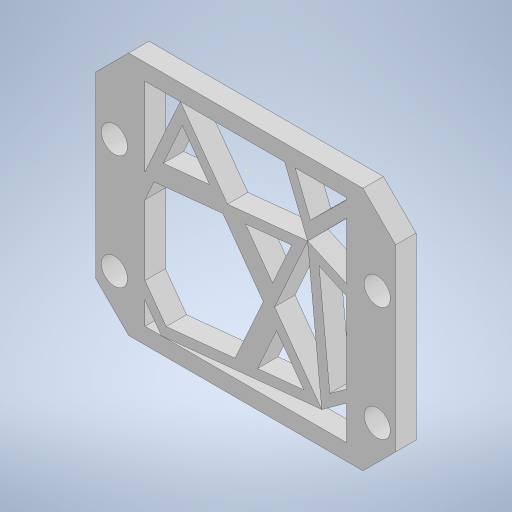
# Autodesk Inventor part: 1министена
Saved by Autodesk Inventor 2023.1 (Build 271208000, 208)
## iProperties
Created: 2025-12-15
Part Number: 1министена
Material: Типовые
Document SubType Name: Modeling
Designer: DELL
Density: 1 g/cm^3
Appearance: По умолчанию
Author: DELL
Autodesk Inventor part; units mm, degrees
ref_plane "YZ Plane" through (0, 0, 0) normal (1, 0, 0) x (0, 1, 0)
ref_plane "XZ Plane" through (0, 0, 0) normal (0, 1, 0) x (-1, 0, 0)
ref_plane "XY Plane" through (0, 0, 0) normal (0, 0, 1) x (1, 0, 0)
sketch "Эскиз1" plane through (0, 0, 0) normal (0, 0, 1) x (1, 0, 0)
  line L0 (18.0359, -24.7333) -> (-18.1641, -24.7333)
  line L1 (-10.3906, -22.7523) -> (-12.4141, -19.9485)
  line L2 (-12.4141, -6.4014) -> (-12.1226, -5.7523)
  line L3 (-12.1226, -5.7523) -> (-2.3077, -4.7523)
  line L4 (-2.3077, -4.7523) -> (3.4658, -12.7523)
  line L5 (3.4658, -12.7523) -> (-0.5756, -21.7523)
  line L6 (-0.5756, -21.7523) -> (-10.3906, -22.7523)
  line L7 (-1.3865, -20.6287) -> (2.0873, -12.8928)
  line L8 (2.0873, -12.8928) -> (-2.8753, -6.0164)
  line L9 (-2.8753, -6.0164) -> (-11.3118, -6.8759)
  line L10 (-11.3118, -6.8759) -> (-12.4141, -9.3307)
  line L11 (-12.4141, -17.8979) -> (-9.823, -21.4883)
  line L12 (-9.823, -21.4883) -> (-1.3865, -20.6287)
  line L13 (-0.5756, -21.7523) -> (9.2393, -20.7523)
  line L14 (9.2393, -20.7523) -> (3.4658, -12.7523)
  line L15 (7.0499, -19.7692) -> (1.3705, -20.3478)
  line L16 (3.7091, -15.14) -> (1.3705, -20.3478)
  line L17 (3.7091, -15.14) -> (7.0499, -19.7692)
  line L18 (-12.1226, -5.7523) -> (-8.0812, 3.2477)
  line L19 (-8.0812, 3.2477) -> (-2.3077, -4.7523)
  line L20 (-2.3077, -4.7523) -> (-12.1226, -5.7523)
  line L21 (-10.1765, -4.3478) -> (-4.4971, -3.7692)
  line L22 (-4.4971, -3.7692) -> (-7.8379, 0.86)
  line L23 (-7.8379, 0.86) -> (-10.1765, -4.3478)
  line L24 (3.4658, -12.7523) -> (-2.3077, -4.7523)
  line L25 (-2.3077, -4.7523) -> (7.5073, -3.7523)
  line L26 (7.5073, -3.7523) -> (3.4658, -12.7523)
  line L27 (-0.1183, -5.7355) -> (5.5611, -5.1568)
  line L28 (5.5611, -5.1568) -> (3.2226, -10.3647)
  line L29 (-0.1183, -5.7355) -> (3.2226, -10.3647)
  line L30 (7.5073, -3.7523) -> (4.6974, 3.2477)
  line L31 (12.2859, 1.0617) -> (7.5073, -3.7523)
  line L32 (12.2859, 3.0053) -> (7.8466, -1.3764)
  line L33 (7.8466, -1.3764) -> (5.9905, 3.2477)
  line L34 (7.5073, -3.7523) -> (9.2393, -20.7523)
  line L35 (9.2393, -20.7523) -> (11.4529, -19.1548)
  line L36 (7.5073, -3.7523) -> (12.2859, -5.8982)
  line L37 (8.9118, -5.6985) -> (12.2859, -7.2136)
  line L38 (10.2225, -18.5629) -> (12.2859, -17.0738)
  line L39 (8.9118, -5.6985) -> (10.2225, -18.5629)
  line L40 (-5.1674, 3.2477) -> (-5.2923, 2.7696)
  line L41 (-5.2923, 2.7696) -> (-7.3317, 2.2091)
  line L42 (-9.7892, 3.2477) -> (-8.6058, 2.0793)
  line L43 (-18.1641, -24.7333) -> (18.2859, -24.7333)
  line L44 (18.0359, 5.2287) -> (-18.1641, 5.2287)
  line L45 (-18.1641, -24.7333) -> (18.0359, 5.2287) construction
  line L46 (18.2859, 5.2287) -> (-18.4141, 5.2287)
  line L47 (-18.4141, 5.2287) -> (-18.4141, -24.7333)
  line L48 (-18.4141, -24.7333) -> (18.2859, -24.7333)
  line L49 (18.2859, -24.7333) -> (18.2859, 5.2287)
  line L50 (18.2859, 5.2287) -> (-18.4141, -24.7333) construction
  line L51 (-18.4141, 5.2287) -> (18.2859, -24.7333) construction
  line L52 (14.0359, 3.2477) -> (-14.1641, -22.7523) construction
  line L53 (-14.1641, 3.2477) -> (14.0359, -22.7523) construction
  line L54 (12.2859, 3.2477) -> (-12.4141, 3.2477)
  line L55 (-12.4141, 3.2477) -> (-12.4141, -22.7523)
  line L56 (-12.4141, -22.7523) -> (12.2859, -22.7523)
  line L57 (12.2859, -22.7523) -> (12.2859, 3.2477)
  line L58 (12.2859, 3.2477) -> (-12.4141, -22.7523) construction
  line L59 (-12.4141, 3.2477) -> (12.2859, -22.7523) construction
  line L60 (11.4529, -19.1548) -> (12.2859, -18.5536)
  point P0 (0, 0)
  point P1 (-6.3491, -13.7523)
  point P2 (-7.5038, -2.419)
  point P3 (2.8885, -7.0857)
  point P4 (-0.0641, -9.7523)
  point P5 (18.0359, 5.2287)
  dimension "d22" = 1.2
  dimension "d25" = 9
  dimension "d26" = 60
  dimension "d27" = 60
  dimension "d31" = 1.2
  dimension "d32" = 1.2
  dimension "d33" = 1.2
  dimension "d39" = 1.2
  dimension "d40" = 1.2
  dimension "d41" = 1.2
  dimension "d44" = 1.2
  dimension "d45" = 1.2
  dimension "d46" = 1.2
  dimension "d75" = 60
  dimension "d76" = 60
  dimension "d77" = 1.2
  dimension "d79" = 1.2
  dimension "d81" = 1.2
  dimension "d84" = 1.2
  dimension "d137" = 24.7
  dimension "d138" = 6
  dimension "d139" = 29.962
  constraints: 122 end point, 15 point on line, 12 parallel, 7 midpoint, 3 horizontal, 2 perpendicular, 27 other
  measures "d22" distance between parallel lines of L5 L7
  measures "d25" vertical distance of L4.end L5.end
  measures "d26" angle of L5 L14
  measures "d27" angle of L5 L13
  measures "d31" distance between parallel lines of L14 L17
  measures "d32" distance between parallel lines of L13 L15
  measures "d33" distance between parallel lines of L5 L16
  measures "d39" distance between parallel lines of L19 L22
  measures "d40" distance between parallel lines of L18 L23
  measures "d41" distance between parallel lines of L3 L21
  measures "d44" distance between parallel lines of L25 L27
  measures "d45" distance between parallel lines of L26 L28
  measures "d46" distance between parallel lines of L4 L29
  measures "d75" angle of L34 L35
  measures "d76" angle of L34 L36
  measures "d77" distance between parallel lines of L36 L37
  measures "d79" distance between parallel lines of L35 L38
  measures "d81" distance between parallel lines of L34 L39
  measures "d84" distance between parallel lines of L30 L33
  measures "d137" distance of L56.end L55.end
  measures "d138" distance between parallel lines of L47 L55
  measures "d139" distance of L43.end L46.start
extrude "Выдавливание1" add sketch "Эскиз1" along normal blind 2.5 contours L0 L48 L47 L46 L44 L49 L43 | L1 L55 L11 L12 L7 L8 L9 L10 L2 L3 L4 L5 L6 | L5 L14 L13 | L4 L25 L26 | L34 L36 L57 L37 L39 L38 L60 L35 | L3 L18 L19 | L30 L54 L33 L32 L57 L31
sketch "Эскиз2" plane through (0, 0, 2.5) normal (0, 0, 1) x (1, 0, 0)
  circle A0 centre (-16.1641, -4.7713) radius 1.6
  line L0 (-14.1641, -6.4014) -> (-14.1641, 3.2477) projected
  line L1 (18.2859, 5.2287) -> (-18.4141, 5.2287) projected
  circle A1 centre (-16.1641, -18.7713) radius 1.6
  line L2 (-0.0641, 5.2287) -> (-0.0641, -30.3358) construction
  circle A2 centre (16.0359, -4.7713) radius 1.6
  circle A3 centre (16.0359, -18.7713) radius 1.6
  point P0 (0, 0)
  point P1 (-12.4141, -6.4014)
  point P2 (-14.1641, 3.2477)
  dimension "d124" = 3.2
  dimension "d125" = 2
  dimension "d126" = 10
  dimension "d127" = 3.2
  dimension "d128" = 14
  constraints: 4 centre point, 2 end point, 2 symmetric about line, 1 midpoint, 1 vertical, 2 other
  measures "d124" diameter of A0
  measures "d125" distance from line of L0 A0.centre
  measures "d126" distance from line of L1 A0.centre
  measures "d127" diameter of A1
  measures "d128" distance of A0.centre A1.centre
extrude "Выдавливание2" cut sketch "Эскиз2" against normal blind 2.5
chamfer "Фаска1" distance 4 angle 45 4 edges at (-18.4141, 5.2287, 1.25) (18.2859, 5.2287, 1.25) (-18.4141, -24.7333, 1.25) (18.2859, -24.7333, 1.25)
sketch "Эскиз3" plane through (0, 0, 2.5) normal (0, 0, 1) x (1, 0, 0)
  point P0 (0, 0)
